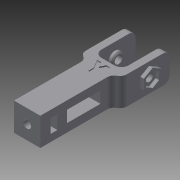
# Autodesk Inventor part: x_tensioner
Saved by Autodesk Inventor 2014 (Build 180170000, 170)
## iProperties
Created: 2016-05-12
Part Number: x_tensioner
Material: Generic
Document SubType Name: Modeling
Designer: 101767
Density: 1 g/cm^3
Appearance: Default
Author: 101767
Autodesk Inventor part; units mm, degrees
ref_plane "XZ Plane" through (0, 0, 0) normal (0, 1, 0) x (-1, 0, 0)
ref_plane "XY Plane" through (0, 0, 0) normal (0, 0, 1) x (1, 0, 0)
sketch "Sketch1" plane through (0, 0, 0) normal (0, 0, 1) x (1, 0, 0)
  line L0 (0, -10.6) -> (0, 63.6) construction
  line L1 (0, 0) -> (-5.7, 0)
  line L2 (-5.7, 0) -> (-5.7, 32)
  line L3 (-5.7, 32) -> (-8.9, 32)
  line L4 (-8.9, 32) -> (-8.9, 53)
  line L5 (-8.9, 53) -> (-5.9, 53)
  line L6 (-5.9, 35) -> (0, 35)
  line L7 (-13.997, 44) -> (0, 44) construction
  line L8 (-5.9, 53) -> (-5.9, 35)
  line L9 (0, 0) -> (5.7, 0)
  line L10 (5.7, 0) -> (5.7, 32)
  line L11 (5.7, 32) -> (8.9, 32)
  line L12 (8.9, 32) -> (8.9, 53)
  line L13 (8.9, 53) -> (5.9, 53)
  line L14 (5.9, 35) -> (0, 35)
  line L15 (13.997, 44) -> (0, 44) construction
  line L16 (5.9, 53) -> (5.9, 35)
  dimension "d6" = 32
  dimension "d7" = 3
  dimension "d8" = 3
  dimension "d9" = 5.7
  dimension "d10" = 18
  dimension "d12" = 9
  dimension "d19" = 5.9
  constraints: 32 end point, 7 symmetric about line, 4 parallel, 4 perpendicular, 3 point on line
  measures "d6" distance of L1.end L2.end
  measures "d7" distance of L4.end L5.end
  measures "d8" distance between parallel lines of L3 L6
  measures "d9" distance of L1.start L1.end
  measures "d10" distance of L5.end L6.start
  measures "d12" distance between parallel lines of L6 L7
  measures "d19" distance between parallel lines of L0 L8
extrude "Extrusion1" add sketch "Sketch1" along normal blind 12.1
ref_plane "Work Plane1" through (4.4, 0, 0) normal (1, 0, 0) x (0, 1, 0)
sketch "Sketch2" plane through (4.4, 0, 0) normal (1, 0, 0) x (0, 1, 0)
  line L0 (35, 0) -> (35, 12.1) construction
  line L1 (53, 0) -> (53, 12.1) construction
  line L2 (35, 6.05) -> (53, 6.05) construction
  circle A0 centre (44, 6.05) radius 2.75
  line L3 (44, -3.8243) -> (44, 13.7141) construction
  line L4 (35, 0) -> (53, 0) construction
  line L5 (53, 12.1) -> (35, 12.1) construction
  point P0 (0, 0)
  dimension "d21" = 5.5
  dimension "d22" = 18
  dimension "d23" = 9
  constraints: 4 end point, 3 midpoint, 1 centre point, 1 perpendicular, 1 point on line
  measures "d21" diameter of A0
  measures "d22" distance between parallel lines of L1 L0
  measures "d23" distance between parallel lines of L0 L3
extrude "Extrusion2" add sketch "Sketch2" along normal up to next
chamfer "Chamfer1" distance 0.5 angle 45 1 edges at (4.4, 41.25, 6.05)
mirror "Mirror1" about plane through (0, 0, 0) normal (1, 0, 0) of "Extrusion2", "Chamfer1"
sketch "Sketch3" plane through (0, 0, 0) normal (1, 0, 0) x (0, 1, 0)
  circle A0 centre (44, 6.05) radius 2.75 construction
  circle A1 centre (44, 6.05) radius 1.65
  point P0 (0, 0)
  dimension "d26" = 3.3
  constraints: 1 centre point, 1 coincident
  measures "d26" diameter of A1
extrude "Extrusion3" cut sketch "Sketch3" along normal through all both and the other way through all
fillet "Fillet1" radius 3 10 edges at (5.9, 35, 6.05) (8.9, 32, 6.05) (-5.7, 32, 6.05) (5.7, 32, 6.05) (-8.9, 32, 6.05) (-5.9, 35, 6.05) (-7.4, 53, 12.1) (7.4, 53, 12.1) (7.4, 53, 0) (-7.4, 53, 0)
sketch "Sketch4" plane through (0, 0, 0) normal (1, 0, 0) x (0, 1, 0)
  line L0 (26.0923, 3.55) -> (11.5923, 3.55)
  line L1 (11.5923, 3.55) -> (11.5923, 6.05)
  line L2 (11.5923, 8.55) -> (26.0923, 8.55)
  line L3 (26.0923, 8.55) -> (26.0923, 3.55)
  line L4 (0, 12.1) -> (29, 12.1) construction
  line L5 (29, 0) -> (0, 0) construction
  line L6 (0, 0) -> (0, 12.1) construction
  line L7 (29, 6.05) -> (-2.186, 6.05) construction
  line L8 (11.5923, 6.05) -> (11.5923, 8.55)
  dimension "d33" = 5
  dimension "d34" = 12.1
  dimension "d35" = 6.05
  dimension "d36" = 2.5
  dimension "d37" = 14.5
  constraints: 12 end point, 3 parallel, 3 perpendicular, 1 horizontal, 1 point on line
  measures "d33" distance of L0.end L2.start
  measures "d34" distance between parallel lines of L5 L4
  measures "d35" distance between parallel lines of L5 L7
  measures "d36" distance of L0.end L1.end
  measures "d37" distance of L2.start L2.end
extrude "Extrusion4" cut sketch "Sketch4" along normal through all both and the other way through all
sketch "Sketch5" plane through (5.7, 0, 12.1) normal (1, 0, 0) x (0, 0, -1)
  line L0 (0, 0) -> (0, 29) construction
  line L1 (12.1, 0) -> (0, 0) construction
  line L2 (12.1, 29) -> (12.1, 0) construction
  line L3 (9.05, 4.5) -> (3.05, 4.5)
  line L4 (3.05, 4.5) -> (3.05, 7.4)
  line L5 (3.05, 7.4) -> (9.05, 7.4)
  line L6 (9.05, 7.4) -> (9.05, 4.5)
  line L7 (6.05, 28.3578) -> (6.05, -4.0028) construction
  dimension "d40" = 6
  dimension "d41" = 2.9
  dimension "d42" = 12.1
  dimension "d43" = 6.05
  dimension "d44" = 3
  dimension "d45" = 4.5
  constraints: 10 end point, 3 parallel, 1 horizontal, 1 perpendicular
  measures "d40" distance of L4.end L5.end
  measures "d41" distance of L5.end L3.start
  measures "d42" distance between parallel lines of L2 L0
  measures "d43" distance between parallel lines of L0 L7
  measures "d44" distance between parallel lines of L4 L7
  measures "d45" distance between parallel lines of L1 L3
extrude "Extrusion5" cut sketch "Sketch5" against normal through all
sketch "Sketch6" plane through (-5.7, 0, 0) normal (0, -1, 0) x (1, 0, 0)
  line L0 (11.4, 0) -> (0, 0) construction
  line L1 (0, 0) -> (0, 12.1) construction
  circle A0 centre (5.7, 6.05) radius 1.65
  point P0 (5.7, 0)
  dimension "d48" = 3.3
  dimension "d49" = 11.4
  dimension "d50" = 12.1
  dimension "d51" = 5.7
  dimension "d52" = 6.05
  constraints: 1 centre point
  measures "d48" diameter of A0
  measures "d49" distance of L0.start L0.end
  measures "d50" distance of L0.end L1.end
  measures "d51" distance from line of A0.centre L1
  measures "d52" distance from line of A0.centre L0
extrude "Extrusion6" cut sketch "Sketch6" against normal up to surface (26.0923 mm away)
sketch "Sketch7" plane through (8.9, 34.3066, 0) normal (1, 0, 0) x (0, 0, -1)
  line L0 (-3, 18.6934) -> (-9.1, 18.6934) construction
  circle A0 centre (-6.05, 9.6934) radius 1.65 construction
  line L1 (-4.4334, 12.4934) -> (-2.8168, 9.6934)
  line L2 (-2.8168, 9.6934) -> (-4.4334, 6.8934)
  line L3 (-4.4334, 6.8934) -> (-7.6666, 6.8934)
  line L4 (-7.6666, 6.8934) -> (-9.2832, 9.6934)
  line L5 (-9.2832, 9.6934) -> (-7.6666, 12.4934)
  line L6 (-7.6666, 12.4934) -> (-4.4334, 12.4934)
  line L7 (-3.8561, 13.4934) -> (-1.6621, 9.6934)
  line L8 (-1.6621, 9.6934) -> (-3.8561, 5.8934)
  line L9 (-3.8561, 5.8934) -> (-8.2439, 5.8934)
  line L10 (-8.2439, 5.8934) -> (-10.4379, 9.6934)
  line L11 (-10.4379, 9.6934) -> (-8.2439, 13.4934)
  line L12 (-8.2439, 13.4934) -> (-3.8561, 13.4934)
  point P0 (0, -34.3066)
  dimension "d55" = 5.6
  dimension "d56" = 1
  constraints: 24 end point, 1 coincident, 1 parallel, 18 other
  measures "d55" distance between parallel lines of L3 L6
  measures "d56" distance between parallel lines of L9 L3
extrude "Extrusion7" add sketch "Sketch7" along normal blind 1.5
sketch "Sketch8" plane through (0, 0, 12.1) normal (0, 0, 1) x (1, 0, 0)
  line L0 (-2.8695, 33.3082) -> (2.9734, 33.3082) construction
  line L1 (2.9734, 33.3082) -> (2.9734, 27.2082) construction
  line L2 (2.9734, 27.2082) -> (-2.8695, 27.2082) construction
  line L3 (-2.8695, 27.2082) -> (-2.8695, 33.3082) construction
  line L4 (2.835, 33.3082) -> (0.7292, 29.754)
  line L5 (0.7292, 29.754) -> (0.7292, 27.2082)
  line L6 (0.7292, 27.2082) -> (-0.8032, 27.2082)
  line L7 (-0.8032, 27.2082) -> (-0.8032, 29.6798)
  line L8 (-0.8032, 29.6798) -> (-2.9437, 33.3082)
  line L9 (-2.9437, 33.3082) -> (-1.1987, 33.3082)
  line L10 (-1.1987, 33.3082) -> (-0.0074, 31.1331)
  line L11 (-0.0074, 31.1331) -> (1.1444, 33.3082)
  line L12 (1.1444, 33.3082) -> (2.835, 33.3082)
  point P0 (0, 0)
  constraints: 2 other
emboss "Emboss1" sketch "Sketch8" operation cut depth 0.5 direction (0, 0, -1)
equation "\"d23\" = 0.5 * d22"
equation "\"d35\" = 0.5 * d34"
equation "\"d36\" = 0.5 * d33"
equation "\"d43\" = 0.5 * d42"
equation "\"d44\" = 0.5 * d40"
equation "\"d51\" = 0.5 * d49"
equation "\"d52\" = 0.5 * d50"
body "Solid1"
